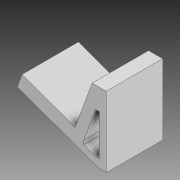
# Autodesk Inventor part: LEDbracket
Saved by Autodesk Inventor 2020 (Build 240168000, 168)
## iProperties
Created: 2021-01-14
Part Number: LEDbracket
Material: Generic
Document SubType Name: Modeling
Designer: DDeGo
Density: 1 g/cm^3
Appearance: Default
Author: DDeGo
Autodesk Inventor part; units mm, degrees
ref_plane "YZ Plane" through (0, 0, 0) normal (1, 0, 0) x (0, 1, 0)
ref_plane "XZ Plane" through (0, 0, 0) normal (0, 1, 0) x (-1, 0, 0)
ref_plane "XY Plane" through (0, 0, 0) normal (0, 0, 1) x (1, 0, 0)
sketch "Sketch1" plane through (0, 0, 0) normal (0, 0, 1) x (1, 0, 0)
  line L0 (0, 0) -> (1, 0)
  line L1 (1, 0) -> (1, 10)
  line L2 (1, 10) -> (-1, 10)
  line L3 (-1, 10) -> (-3.4129, 3.3706)
  line L4 (-3.4129, 3.3706) -> (-10.9305, 6.1067)
  line L5 (-10.9305, 6.1067) -> (-11.6145, 4.2273)
  line L6 (-11.6145, 4.2273) -> (0, 0)
  line L7 (-0.5, 6.988) -> (-2.1847, 2.3593)
  line L8 (-2.1847, 2.3593) -> (-2.1847, 1.8593)
  line L9 (-2.1847, 1.8593) -> (-0.5, 1.2462)
  line L10 (-0.5, 1.2462) -> (0, 1.2462)
  line L11 (0, 1.2462) -> (0, 6.988)
  line L12 (0, 6.988) -> (-0.5, 6.988)
  dimension "d0" = 70
  dimension "d1" = 2
  dimension "d2" = 2
  dimension "d3" = 8
  dimension "d4" = 10
  dimension "d5" = 1
  dimension "d6" = 0.5
  dimension "d7" = 0.5
  dimension "d8" = 0.5
  dimension "d9" = 1
  dimension "d11" = 1.5
  dimension "d12" = 1
  constraints: 26 end point, 6 perpendicular, 4 parallel, 1 horizontal, 1 vertical
  measures "d0" angle of L0 L3
  measures "d1" distance of L1.end L2.end
  measures "d2" distance between parallel lines of L6 L4
  measures "d3" distance of L3.end L4.end
  measures "d4" distance of L0.end L1.end
  measures "d5" distance of L0.start L0.end
  measures "d6" distance of L11.end L7.start
  measures "d7" distance of L7.end L8.end
  measures "d8" distance of L9.end L10.end
  measures "d9" distance between parallel lines of L1 L11
  measures "d11" distance between parallel lines of L3 L7
  measures "d12" distance between parallel lines of L6 L9
extrude "Extrusion1" add sketch "Sketch1" along normal mid plane 8
body "Solid1"
